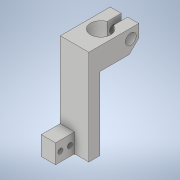
# Autodesk Inventor part: MEM to dovetail rod adapter - v3
Saved by Autodesk Inventor 2021 (Build 250183000, 183)
## iProperties
Created: 2020-08-03
Part Number: MEM to dovetail rod adapter - v3
Material: Generic
Document SubType Name: Modeling
Designer: eric
Density: 1 g/cm^3
Appearance: Default
Author: eric
Autodesk Inventor part; units mm, degrees
ref_plane "YZ Plane" through (0, 0, 0) normal (1, 0, 0) x (0, 1, 0)
ref_plane "XZ Plane" through (0, 0, 0) normal (0, 1, 0) x (-1, 0, 0)
sketch "Sketch1" plane through (0, 0, 0) normal (1, 0, 0) x (0, 1, 0)
  line L0 (0, 0) -> (30, 0)
  line L1 (30, 0) -> (30, -3.5)
  line L2 (30, -3.5) -> (0, -3.5)
  line L3 (0, -3.5) -> (0, 0)
  dimension "d0" = 3.5
  dimension "d1" = 30
  constraints: 8 end point, 2 parallel, 1 horizontal, 1 perpendicular
  measures "d0" distance of L0.end L1.end
  measures "d1" distance of L1.end L2.end
extrude "Extrusion1" add sketch "Sketch1" along normal mid plane 9
sketch "Sketch2" plane through (-4.5, 0, -3.5) normal (0, 0, -1) x (-1, 0, 0)
  line L0 (-9, 30) -> (0, 30) projected
  line L1 (0, 0) -> (0, 30) projected
  line L2 (-9, 30) -> (0, 30)
  line L3 (0, 30) -> (0, 23)
  line L4 (0, 23) -> (-9, 23)
  line L5 (-9, 23) -> (-9, 30)
  point P0 (-4.5, 0)
  dimension "d4" = 7
  constraints: 8 end point, 2 parallel, 1 horizontal, 1 perpendicular, 2 other
  measures "d4" distance between parallel lines of L0 L4
extrude "Extrusion2" add sketch "Sketch2" along normal blind 12.25
ref_plane "Work Plane1" through (0, 0, 0) normal (-1, 0, 0) x (0, 0, 1)
sketch "Sketch3" plane through (-4.5, 0, 0) normal (0, 0, 1) x (1, 0, 0)
  line L0 (4.5, 0) -> (9, 0) projected
  line L1 (0, 0) -> (4.5, 0)
  line L2 (4.5, 0) -> (4.5, 6)
  line L3 (4.5, 6) -> (0, 6)
  line L4 (0, 6) -> (0, 0)
  line L5 (9, 30) -> (0, 30) projected
  line L6 (4.5, -6) -> (4.5, 36) projected
  point P0 (4.5, 30)
  dimension "d7" = 4.5
  dimension "d8" = 4.5
  dimension "d9" = 6
  constraints: 8 end point, 2 parallel, 1 horizontal, 1 midpoint, 1 perpendicular, 1 point on line
  measures "d7" distance between parallel lines of L6 L4
  measures "d8" distance of L2.end L3.end
  measures "d9" distance of L3.end L1.start
extrude "Extrusion3" add sketch "Sketch3" along normal blind 6
sketch "Sketch7" plane through (-4.5, 30, 0) normal (0, 1, 0) x (1, 0, 0)
  circle A0 centre (4.5, 8.25) radius 3.2004
  line L0 (0, 15.75) -> (9, 15.75) projected
  point P0 (4.5, 0)
  dimension "d42" = 6.4008
  dimension "d43" = 7.5
  constraints: 1 centre point
  measures "d42" diameter of A0
  measures "d43" distance from line of L0 A0.centre
extrude "Extrusion6" cut sketch "Sketch7" against normal up to next
sketch "Sketch8" plane through (-4.5, 30, 0) normal (0, 1, 0) x (1, 0, 0)
  line L0 (9, 15.75) -> (0, 15.75) projected
  line L1 (5.5, 7.75) -> (3.5, 7.75)
  line L2 (3.5, 7.75) -> (3.5, 15.75)
  line L3 (3.5, 15.75) -> (5.5, 15.75)
  line L4 (5.5, 15.75) -> (5.5, 7.75)
  line L5 (5.5, 7.75) -> (3.5, 15.75) construction
  line L6 (3.5, 7.75) -> (5.5, 15.75) construction
  line L7 (4.5, -3.15) -> (4.5, 18.9) projected
  point P0 (4.5, 0)
  point P1 (4.5, 11.75)
  dimension "d46" = 8
  dimension "d47" = 2
  dimension "d48" = 1
  constraints: 12 end point, 2 midpoint, 2 parallel, 1 horizontal, 1 perpendicular, 1 point on line
  measures "d46" distance of L1.end L2.end
  measures "d47" distance between parallel lines of L4 L2
  measures "d48" distance between parallel lines of L7 L2
extrude "Extrusion7" cut sketch "Sketch8" against normal up to next
sketch "Sketch9" plane through (4.5, 0, 0) normal (1, 0, 0) x (0, 0, -1)
  line L0 (0, 30) -> (15.75, 30) projected
  line L1 (15.75, 30) -> (15.75, 23) projected
  point P0 (0, 0)
  point P1 (13.25, 27)
  dimension "d51" = 3
  dimension "d52" = 2.5
  measures "d51" distance from line of L0 point (13.25, 27)
  measures "d52" distance from line of L1 point (13.25, 27)
hole "Hole2" at (4.5, 27, -13.25) direction (-1, 0, 0) diameter 3.4 depth 3.5 clearance for "Flat Head Machine Screw" size "M3" standard "Ansi Metric M Profile"
sketch "Sketch10" plane through (-1, 30, -11.2902) normal (1, 0, 0) x (0, 0, -1)
  circle A0 centre (1.9598, -3) radius 1.7 projected
  point P0 (-11.2902, -30)
  point P1 (3.0161, 3.0772)
  constraints: 1 coincident
hole "Hole3" at (-1, 27, -13.25) direction (-1, 0, 0) diameter 2.459 depth 3.5 thread size "M3x0.5" class "6H" standard "ANSI Metric M Profile"
chamfer "Chamfer1" distance 3 angle 45 2 edges at (2.75, 23, -15.75) (-2.75, 23, -15.75)
sketch "Sketch13" plane through (0, 0, 0) normal (1, 0, 0) x (0, 0, -1)
  line L0 (0, 0) -> (-6, 0) projected
  line L1 (-6, 0) -> (-6, 6) projected
  line L2 (0, 6) -> (-6, 6) projected
  line L3 (0, 30) -> (0, 0) projected
  point P0 (-4.5, 3)
  dimension "d91" = 3
  dimension "d92" = 4.5
  measures "d91" distance from line of L2 point (-4.5, 3)
  measures "d92" distance from line of L3 point (-4.5, 3)
hole "Hole4" at (0, 3, 4.5) direction (-1, 0, 0) diameter 1.567 end through all thread size "M2x0.4" class "6H" standard "ANSI Metric M Profile"
sketch "Sketch14" plane through (0, 0, 0) normal (1, 0, 0) x (0, 0, -1)
  line L0 (-6, 0) -> (-6, 6) projected
  line L1 (0, 6) -> (-6, 6) projected
  point P0 (0, 0)
  point P1 (-1.5, 3)
  dimension "d100" = 4.5
  dimension "d101" = 3
  measures "d100" distance from line of L0 point (-1.5, 3)
  measures "d101" distance from line of L1 point (-1.5, 3)
hole "Hole5" at (0, 3, 1.5) direction (-1, 0, 0) diameter 1.567 end through all thread size "M2x0.4" class "6H" standard "ANSI Metric M Profile"
body "Solid1"
